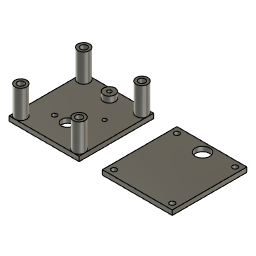
GearTestBox (Autodesk Fusion 360 design; units mm, degrees)
Autodesk Fusion 360 part; units mm, degrees
note: some values were not read from the file. Set by a fixed rule: which sketch regions a step uses.
sketch "Sketch1" plane through (0, 0, 0) normal (0, 0, 1) x (1, 0, 0)
  line L0 (0, 0) -> (38.1, 0)
  line L1 (38.1, 0) -> (38.1, 40.64)
  line L2 (38.1, 40.64) -> (0, 40.64)
  line L3 (0, 40.64) -> (0, 0)
  dimension "d1" = 38.1
  dimension "d2" = 40.64
  constraint horizontal L0
  constraint vertical L1
  constraint horizontal L2
  constraint vertical L3
  constraint coincident L0.start L3.end
  measures "d1" distance of L0.start L0.end
  measures "d2" distance of L0.start L2.end
  measures "d9" distance of L0.start
  measures "d14" distance of L0.start
  measures "d15" distance of L0.start
extrude "Extrude1" add sketch "Sketch1" along normal blind 2.54 makes body 1
sketch "Sketch2" plane through (0, 0, 2.54) normal (0, 0, 1) x (-1, 0, 0)
  line L0 (0, -40.64) -> (0, 0)
  line L1 (0, 0) -> (-38.1, 0)
  line L2 (-38.1, 0) -> (-38.1, -40.64)
  line L3 (-38.1, -40.64) -> (0, -40.64)
  circle A0 centre (-19.05, -12.7) radius 3.175
  circle A1 centre (-12.0523, -12.7) radius 1.27
  circle A2 centre (-26.0477, -12.7) radius 1.27
  circle A3 centre (-27.94, -24.13) radius 1.0655
  circle A4 centre (-19.05, -35.56) radius 1.0655
  circle A5 centre (-19.05, -35.56) radius 3.175
  dimension "d5" = 6.35
  dimension "d6" = 2.54
  dimension "d7" = 2.54
  dimension "d8" = 13.9954
  dimension "d9" = 12.7
  dimension "d10" = 12.0523
  dimension "d11" = 2.1311
  dimension "d12" = 2.1311
  dimension "d13" = 8.89
  dimension "d14" = 11.43
  dimension "d15" = 19.05
  dimension "d16" = 22.86
  dimension "d18" = 6.35
  constraint horizontal A0.centre A1.centre
  constraint horizontal A0.centre A2.centre
  constraint concentric A4 A5
  measures "d5" diameter of A0
  measures "d6" diameter of A1
  measures "d7" diameter of A2
  measures "d8" distance of A1.centre A2.centre
  measures "d9" distance of L1 A0.centre
  measures "d10" distance of L0 A1.centre
  measures "d11" diameter of A3
  measures "d12" diameter of A4
  measures "d13" horizontal distance of A0.centre A3.centre
  measures "d14" vertical distance of A0.centre A3.centre
  measures "d15" distance of L2 A4.centre
  measures "d16" distance of A0.centre A4.centre
  measures "d18" diameter of A5
extrude "Extrude2" cut sketch "Sketch2" against normal blind 2.54 contours A0 | A1 | A2 | A3 | A4 bodies 1
extrude "Extrude3" add sketch "Sketch2" along normal blind 3.302 contours A5 bodies 1
chamfer "Chamfer1" distance 1.016 angle 55 1 edges at (22.0101, 34.4119, 2.54) measured on face at (9.2813, 29.4038, 2.54) on bodies 1
delete_face "DeleteFace1" 1 faces at (20.4574, 39.146, 3.0237) on bodies 1
sketch "Sketch3" plane through (0, 0, 2.54) normal (0, 0, 1) x (-1, 0, 0)
  circle A0 centre (-19.05, -35.56) radius 3.175
  line L0 (0, -40.64) -> (0, 0)
  line L1 (0, 0) -> (-38.1, 0)
  line L2 (-38.1, 0) -> (-38.1, -40.64)
  line L3 (-38.1, -40.64) -> (0, -40.64)
  circle A1 centre (-12.0523, -12.7) radius 1.27
  circle A2 centre (-26.0477, -12.7) radius 1.27
  circle A3 centre (-27.94, -24.13) radius 1.0655
  circle A4 centre (-19.05, -12.7) radius 3.175
  circle A5 centre (-3.175, -3.175) radius 3.175
  circle A6 centre (-3.175, -3.175) radius 1.8097
  circle A7 centre (-34.925, -3.175) radius 3.175
  circle A8 centre (-34.925, -3.175) radius 1.8097
  circle A9 centre (-3.175, -37.465) radius 3.175
  circle A10 centre (-3.175, -37.465) radius 1.8097
  circle A11 centre (-34.925, -37.465) radius 3.175
  circle A12 centre (-34.925, -37.465) radius 1.8097
  dimension "d25" = 6.35
  dimension "d26" = 3.6195
  dimension "d29" = -31.75
  dimension "d30" = -34.29
  dimension "d53" = 3.175
  dimension "d54" = 3.175
  constraint concentric A5 A6
  measures "d25" diameter of A5
  measures "d26" diameter of A6
  measures "d53" distance of L1 A5.centre
  measures "d54" distance of L0 A5.centre
extrude "Extrude4" add sketch "Sketch3" along normal blind 16.51 contours A9 | A5 | A11 | A7 bodies 1
extrude "Extrude5" add 4 faces at (33.8233, 3.5148, 2.54) (34.7908, 38.0531, 2.54) (3.3092, 36.8769, 2.54) (2.5874, 3.5283, 2.54) along direction (0, 0, 1) blind 12.5095 on bodies 1 bodies 1
sketch "Sketch4" plane through (0, 0, 0) normal (0, 0, 1) x (1, 0, 0)
  line L0 (50.8, 0) -> (88.9, 0)
  line L1 (88.9, 0) -> (88.9, 40.64)
  line L2 (88.9, 40.64) -> (50.8, 40.64)
  line L3 (50.8, 40.64) -> (50.8, 0)
  dimension "d35" = 38.1
  dimension "d36" = 40.64
  constraint horizontal L0
  constraint vertical L1
  constraint horizontal L2
  constraint vertical L3
  measures "d35" distance of L0.start L0.end
  measures "d36" distance of L0.start L2.end
extrude "Extrude6" add sketch "Sketch4" along normal blind 2.54 separate body makes body 2
sketch "Sketch5" plane through (0, 0, 2.54) normal (0, 0, 1) x (-1, 0, 0)
  line L0 (-50.8, -40.64) -> (-50.8, 0)
  line L1 (-50.8, 0) -> (-88.9, 0)
  line L2 (-88.9, 0) -> (-88.9, -40.64)
  line L3 (-88.9, -40.64) -> (-50.8, -40.64)
  circle A0 centre (-53.975, -3.175) radius 1.397
  circle A1 centre (-69.85, -35.56) radius 3.937
  circle A2 centre (-85.725, -3.175) radius 1.397
  circle A3 centre (-53.975, -37.465) radius 1.397
  circle A4 centre (-85.725, -37.465) radius 1.397
  dimension "d39" = 2.794
  dimension "d43" = 7.874
  dimension "d44" = 35.56
  dimension "d55" = 3.175
  dimension "d56" = 3.175
  dimension "d59" = -31.75
  dimension "d60" = -34.29
  measures "d39" diameter of A0
  measures "d43" diameter of A1
  measures "d44" distance of L1 A1.centre
  measures "d55" distance of L1 A0.centre
  measures "d56" distance of L0 A0.centre
extrude "Extrude7" cut sketch "Sketch5" against normal blind 2.54 contours A1 bodies 2
extrude "Extrude8" add sketch "Sketch5" along normal blind 4.0005 contours A0 bodies 2
extrude "Extrude9" cut 4 faces at (0.4669, 3.0173, 19.05) (32.2236, 37.2174, 19.05) (32.2169, 3.0173, 19.05) (0.4669, 37.3073, 19.05) along direction (0, 0, -1) blind 1.27 on bodies 1 bodies 1
extrude "Extrude10" cut 4 faces at (34.7908, 38.0531, 15.0495) (33.8233, 3.5148, 15.0495) (2.5874, 3.5283, 15.0495) (3.3092, 36.8769, 15.0495) along direction (0, 0, -1) blind 1.27 on bodies 1 bodies 1
extrude "Extrude11" cut sketch "Sketch5" against normal blind 11.43 from surface at 5.08 contours A0 | A2 | A3 | A4 bodies 2
